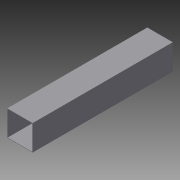
# Autodesk Inventor part: Side Rail
Saved by Autodesk Inventor 2015 SP1 (Build 190203100, 203)
## iProperties
Created: 2016-02-22
Part Number: Side Rail
Material: Generic
Document SubType Name: Modeling
Designer: jonesdm
Density: 1 g/cm^3
Appearance: Default
Author: jonesdm
Autodesk Inventor part; units mm, degrees
ref_plane "YZ Plane" through (0, 0, 0) normal (1, 0, 0) x (0, 1, 0)
ref_plane "XZ Plane" through (0, 0, 0) normal (0, 1, 0) x (-1, 0, 0)
ref_plane "XY Plane" through (0, 0, 0) normal (0, 0, 1) x (1, 0, 0)
sketch "Sketch1" plane through (0, 0, 0) normal (0, 0, 1) x (1, 0, 0)
  line L0 (-25.4, 25.4) -> (25.4, 25.4)
  line L1 (25.4, 25.4) -> (25.4, -25.4)
  line L2 (25.4, -25.4) -> (-25.4, -25.4)
  line L3 (-25.4, -25.4) -> (-25.4, 25.4)
  line L4 (24.638, 24.638) -> (-24.638, 24.638)
  line L5 (-24.638, 24.638) -> (-24.638, -24.638)
  line L6 (-24.638, -24.638) -> (24.638, -24.638)
  line L7 (24.638, -24.638) -> (24.638, 24.638)
  point P0 (0, 0)
  point P1 (0, 25.4)
  point P2 (25.4, 0)
  dimension "d0" = 50.8
  dimension "d1" = 50.8
  dimension "d2" = 0.762
  constraints: 16 end point, 4 parallel, 2 midpoint, 2 perpendicular, 1 horizontal, 1 horizontal alignment, 1 vertical alignment, 3 other
  measures "d0" distance of L0.start L0.end
  measures "d1" distance of L0.end L1.end
  measures "d2" distance between parallel lines of L1 L7
extrude "Extrusion1" add sketch "Sketch1" along normal blind 279.4
sketch "Sketch2" plane through (25.4, -25.4, 0) normal (1, 0, 0) x (0, 0, -1)
  line L0 (0, 50.8) -> (-279.4, 50.8) projected
  line L1 (-279.4, 0) -> (-228.6, 0)
  line L2 (-228.6, 0) -> (-228.6, 50.8)
  line L3 (-228.6, 50.8) -> (-279.4, 50.8)
  line L4 (-279.4, 50.8) -> (-279.4, 0)
  line L5 (-278.638, 0.762) -> (-229.362, 0.762)
  line L6 (-229.362, 0.762) -> (-229.362, 50.038)
  line L7 (-229.362, 50.038) -> (-278.638, 50.038)
  line L8 (-278.638, 50.038) -> (-278.638, 0.762)
  point P0 (0, 25.4)
  dimension "d5" = 50.8
  dimension "d6" = 0.762
  constraints: 16 end point, 4 parallel, 2 perpendicular, 1 horizontal, 1 point on line, 3 other
  measures "d5" distance of L1.start L1.end
  measures "d6" distance between parallel lines of L5 L1
extrude "Extrusion2" add sketch "Sketch2" along normal blind 88.9
sketch "Sketch3" plane through (0, 0, 279.4) normal (0, 0, 1) x (1, 0, 0)
  point P0 (0, 0)
sketch "Sketch4" plane through (0, 0, 279.4) normal (0, 0, 1) x (1, 0, 0)
  line L0 (-25.4, -25.4) -> (114.3, -25.4) projected
  line L1 (114.3, 25.4) -> (63.5, 25.4)
  line L2 (63.5, 25.4) -> (63.5, -25.4)
  line L3 (63.5, -25.4) -> (114.3, -25.4)
  line L4 (114.3, -25.4) -> (114.3, 25.4)
  line L5 (113.538, 24.638) -> (64.262, 24.638)
  line L6 (64.262, 24.638) -> (64.262, -24.638)
  line L7 (64.262, -24.638) -> (113.538, -24.638)
  line L8 (113.538, -24.638) -> (113.538, 24.638)
  point P0 (0, 0)
  dimension "d9" = 50.8
  dimension "d10" = 0.762
  constraints: 16 end point, 4 parallel, 2 perpendicular, 1 horizontal, 1 point on line, 3 other
  measures "d9" distance of L1.start L1.end
  measures "d10" distance between parallel lines of L8 L4
extrude "Extrusion3" add sketch "Sketch4" along normal blind 177.8
body "Solid1"
